Autodesk Inventor part; units mm, degrees
(part 2 of 2)
  dimension "d18" = 152.4
  constraints: 1 centre point, 1 coincident, 1 other
  measures "d18" diameter of A0
extrude "ExtrusionForText" cut sketch "Sketch5" against normal blind 1.27
sketch "Sketch13" plane through (0, -9.525, 0) normal (0, -1, 0) x (1, 0, 0)
  point P0 (0, 0)
  point P1 (44.45, 0)
  point P2 (22.225, 38.4948)
  point P3 (-22.225, 38.4948)
  point P4 (-44.45, 0)
  point P5 (-22.225, -38.4948)
  point P6 (22.225, -38.4948)
  dimension "d65" = 44.45
  dimension "d68" = 360
  constraints: 7 other
  measures "d65" distance of point (44.45, 0) point (0, 0)
hole "Hole6" at (44.45, -9.525, 0) at (22.225, -9.525, 38.4948) at (-22.225, -9.525, 38.4948) at (-44.45, -9.525, 0) at (-22.225, -9.525, -38.4948) at (22.225, -9.525, -38.4948) direction (0, 1, 0) diameter 6.3246 end through all counterbore diameter 7.0891 counterbore depth 6.1239
fillet "Fillet2" radius 1.27 1 edges at (10.795, -44.525, 0)
sketch "Sketch16" plane through (0, 0, 0) normal (0, 1, 0) x (1, 0, 0)
  point P0 (0, 0)
  point P1 (0, 0)
  constraints: 1 coincident
hole "Hole7" at (0, 0, 0) direction (0, -1, 0) diameter 11.9888 end through all clearance for "Flat Head Machine Screw" size "M10" standard "Ansi Metric M Profile"
sketch "Sketch18" plane through (0, 0, 0) normal (0, 1, 0) x (1, 0, 0)
  line L0 (9.9616, 0) -> (4.9808, -8.627)
  line L1 (4.9808, -8.627) -> (-4.9808, -8.627)
  line L2 (-4.9808, -8.627) -> (-9.9616, 0)
  line L3 (-9.9616, 0) -> (-4.9808, 8.627)
  line L4 (-4.9808, 8.627) -> (4.9808, 8.627)
  line L5 (4.9808, 8.627) -> (9.9616, 0)
  point P0 (0, 0)
  point P1 (0, 0)
  dimension "d104" = 17.254
  constraints: 12 end point, 1 coincident, 1 horizontal, 13 other
  measures "d104" distance between parallel lines of L1 L4
extrude "Extrusion8" cut sketch "Sketch18" against normal blind 33.4
equation "\"d18\" = textDiameter"
equation "\"d0\" = topRadius"
equation "\"d3\" = topThickness"
equation "\"d4\" = depthIntoTripod"
equation "\"depthIntoTripod\" = 35"
equation "\"insertionPointDiameter\" = 25.4"
equation "\"insertionPointRadius\" = 0.5 * insertionPointDiameter"
equation "\"topRadius\" = 0.5 * topDiameter"
equation "\"topThickness\" = 9.525"
equation "\"hexBoltClearance\" = 17.635"
equation "\"totalPartHeight\" = depthIntoTripod + topThickness"
equation "\"hexBoltDepth\" = totalPartHeight - hexBoltSupport"
equation "\"hexBoltSupport\" = 9.525"
equation "\"holeForGearBoxHardware\" = 50.8"
equation "\"depthForGearBoxHardware\" = 6.35"
equation "\"textDiameter\" = 152.4"
equation "\"topDiameter\" = 203.2"
body "Solid1"
